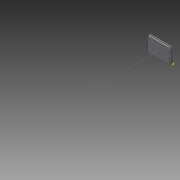
# Autodesk Inventor part: well_plate
Saved by Autodesk Inventor 2015 SP1 (Build 190203100, 203)
## iProperties
Created: 2016-08-02
Part Number: well_plate
Material: Generic
Document SubType Name: Modeling
Designer: polidorop
Density: 1 g/cm^3
Appearance: Default
Author: polidorop
Autodesk Inventor part; units mm, degrees
ref_plane "YZ Plane" through (0, 0, 0) normal (1, 0, 0) x (0, 1, 0)
ref_plane "XZ Plane" through (0, 0, 0) normal (0, 1, 0) x (-1, 0, 0)
ref_plane "XY Plane" through (0, 0, 0) normal (0, 0, 1) x (1, 0, 0)
sketch "Sketch1" plane through (0, 0, 0) normal (0, 0, 1) x (1, 0, 0)
  line L0 (-63.88, 42.74) -> (63.88, 42.74)
  line L1 (63.88, 42.74) -> (63.88, -42.74)
  line L2 (63.88, -42.74) -> (-63.88, -42.74)
  line L3 (-63.88, -42.74) -> (-63.88, 42.74)
  line L4 (63.88, 42.74) -> (-63.88, -42.74) construction
  point P0 (0, 0)
  point P1 (0, 0)
  dimension "d0" = 127.76
  dimension "d1" = 85.48
  constraints: 10 end point, 2 parallel, 1 coincident, 1 horizontal, 1 midpoint, 1 perpendicular
  measures "d0" distance of L0.start L0.end
  measures "d1" distance of L2.end L0.start
extrude "Extrusion1" add sketch "Sketch1" along normal blind 15
sketch "Sketch2" plane through (0, 0, 0) normal (0, 0, -1) x (-1, 0, 0)
  line L0 (-62.7, 41.65) -> (62.7, 41.65)
  line L1 (62.7, 41.65) -> (62.7, -41.65)
  line L2 (62.7, -41.65) -> (-62.7, -41.65)
  line L3 (-62.7, -41.65) -> (-62.7, 41.65)
  line L4 (62.7, 41.65) -> (-62.7, -41.65) construction
  point P0 (0, 0)
  point P1 (0, 0)
  dimension "d4" = 125.4
  dimension "d5" = 83.3
  constraints: 10 end point, 2 parallel, 1 coincident, 1 horizontal, 1 midpoint, 1 perpendicular
  measures "d4" distance of L0.start L0.end
  measures "d5" distance of L2.end L0.start
extrude "Extrusion2" cut sketch "Sketch2" against normal blind 2
sketch "Sketch3" plane through (0, 0, 2) normal (0, 0, -1) x (-1, 0, 0)
  line L0 (-55, 37.5) -> (55, 37.5)
  line L1 (55, 37.5) -> (55, -37.5)
  line L2 (55, -37.5) -> (-55, -37.5)
  line L3 (-55, -37.5) -> (-55, 37.5)
  line L4 (55, 37.5) -> (-55, -37.5) construction
  line L5 (-62.7, 41.65) -> (62.7, 41.65) projected
  line L6 (-62.7, -41.65) -> (-62.7, 41.65) projected
  line L7 (62.7, -41.65) -> (-62.7, -41.65) projected
  line L8 (62.7, 41.65) -> (62.7, -41.65) projected
  point P0 (0, 0)
  point P1 (0, 0)
  dimension "d8" = 75
  dimension "d9" = 110
  constraints: 10 end point, 2 parallel, 1 coincident, 1 horizontal, 1 midpoint, 1 perpendicular
  measures "d8" distance of L0.end L1.end
  measures "d9" distance of L0.start L0.end
extrude "Extrusion3" cut sketch "Sketch3" against normal blind 2
sketch "Sketch4" plane through (0, 0, 15) normal (0, 0, 1) x (1, 0, 0)
  line L0 (61.9, -40.8) -> (-61.9, -40.8)
  line L1 (-61.9, -40.8) -> (-61.9, 40.8)
  line L2 (-61.9, 40.8) -> (61.9, 40.8)
  line L3 (61.9, 40.8) -> (61.9, -40.8)
  line L4 (-61.9, -40.8) -> (61.9, 40.8) construction
  line L5 (63.88, 42.74) -> (-63.88, 42.74) projected
  line L6 (-63.88, 42.74) -> (-63.88, -42.74) projected
  line L7 (-63.88, -42.74) -> (63.88, -42.74) projected
  line L8 (63.88, -42.74) -> (63.88, 42.74) projected
  point P0 (0, 0)
  point P1 (0, 0)
  dimension "d12" = 123.8
  dimension "d13" = 81.6
  constraints: 10 end point, 2 parallel, 1 coincident, 1 horizontal, 1 midpoint, 1 perpendicular
  measures "d12" distance of L0.start L0.end
  measures "d13" distance of L2.end L0.start
extrude "Extrusion4" cut sketch "Sketch4" against normal blind 8.6
fillet "Fillet1" radius 3 8 edges at (62.7, 41.65, 2) (-62.7, 41.65, 2) (-62.7, -41.65, 2) (62.7, -41.65, 2) (63.88, -42.74, 3.2) (63.88, 42.74, 3.2) (-63.88, 42.74, 3.2) (-63.88, -42.74, 3.2)
fillet "Fillet2" radius 2 2 edges at (-61.9, -40.8, 10.7) (-61.9, 40.8, 10.7)
chamfer "Chamfer1" distance 6 angle 45 2 edges at (61.9, -40.8, 10.7) (61.9, 40.8, 10.7)
sketch "Sketch6" plane through (0, 0, 2) normal (0, 0, -1) x (-1, 0, 0)
  circle A0 centre (0, 0) radius 0.5
  dimension "d21" = 1
  constraints: 1 centre point, 1 coincident
  measures "d21" diameter of A0
extrude "Extrusion5" add sketch "Sketch6" against normal blind 800
body "Solid1"
